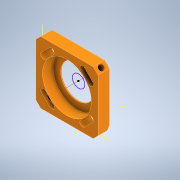
# Autodesk Inventor part: 20_Cube_Insert_Kinematic_Beautymirrormount_90_pro_v3
Saved by Autodesk Inventor 2022.3 (Build 263350000, 350)
## iProperties
Created: 2021-11-15
Part Number: 20_Cube_Insert_Kinematic_Beautymirrormount_90_pro_v3
Material: Generic
Document SubType Name: Modeling
Designer: diederichbenedict
Density: 1 g/cm^3
Appearance: Orange
Author: diederichbenedict
Autodesk Inventor part; units mm, degrees
ref_plane "YZ Plane" through (0, 0, 0) normal (1, 0, 0) x (0, 1, 0)
ref_plane "XY Plane" through (0, 0, 0) normal (0, 0, 1) x (1, 0, 0)
ref_plane "Work Plane1" through (0, 0, 2) normal (0, 0, 1) x (1, 0, 0)
sketch "Sketch1" plane through (0, 0, 2) normal (0, 0, 1) x (1, 0, 0)
  circle A0 centre (-37.0712, 14) radius 3.25 construction
  circle A1 centre (-9.0712, -14) radius 3.25 construction
  line L0 (-26.0712, -17.08) -> (-20.0712, -17.08) construction
  arc A2 (-20.0712, -17.08) -> (-20.0712, -14.08) centre (-20.0712, -15.58) ccw construction
  line L1 (-20.0712, -14.08) -> (-26.0712, -14.08) construction
  line L2 (-37.0712, -3) -> (-37.0712, 3) construction
  arc A3 (-37.0712, 3) -> (-40.0712, 3) centre (-38.5712, 3) ccw construction
  line L3 (-40.0712, 3) -> (-40.0712, -3) construction
  line L4 (-47.9712, -17) -> (-47.9712, 17) construction
  line L5 (-47.9712, 17) -> (-44.3964, 17) construction
  line L6 (-44.3964, 17) -> (-40.0712, 21.3252) construction
  line L7 (-40.0712, 21.3252) -> (-40.0712, 24.9) construction
  line L8 (-40.0712, 24.9) -> (-6.0712, 24.9) construction
  line L9 (-6.0712, 24.9) -> (-6.0712, 21.3252) construction
  line L10 (-6.0712, 21.3252) -> (-1.746, 17) construction
  line L11 (-1.746, 17) -> (1.8288, 17) construction
  line L12 (1.8288, 17) -> (1.8288, -17) construction
  line L13 (1.8288, -17) -> (-1.746, -17) construction
  line L14 (-1.746, -17) -> (-6.1126, -21.3666) construction
  line L15 (-6.1126, -21.3666) -> (-6.1126, -24.9) construction
  line L16 (-6.1126, -24.9) -> (-40.0712, -24.9) construction
  circle A4 centre (-37.0712, -14) radius 3.25 construction
  circle A5 centre (-23.0712, 0) radius 12.45 construction
  circle A6 centre (-23.0712, 0) radius 12.7 construction
  line L17 (-37.0712, 14) -> (-9.0712, 14) construction
  line L18 (-9.0712, 14) -> (-9.0712, -14) construction
  line L19 (-9.0712, -14) -> (-37.0712, -14) construction
  line L20 (-37.0712, -14) -> (-37.0712, 14) construction
  line L21 (-4.0712, -19) -> (-4.0712, 19)
  line L22 (-4.0712, 19) -> (-42.0712, 19)
  line L23 (-42.0712, 19) -> (-42.0712, -19)
  line L24 (-42.0712, -19) -> (-4.0712, -19)
  circle A7 centre (-23.0712, 0) radius 12.8
  circle A8 centre (-23.0712, 0) radius 3.25 projected
  line L25 (-40.0712, -24.9) -> (-40.0712, -21.3252) projected
  line L26 (-40.0712, -21.3252) -> (-44.3964, -17) projected
  line L27 (-44.3964, -17) -> (-47.9712, -17) projected
  arc A9 (-26.0712, -14.08) -> (-26.0712, -17.08) centre (-26.0712, -15.58) ccw projected
  arc A10 (-40.0712, -3) -> (-37.0712, -3) centre (-38.5712, -3) ccw projected
  circle A11 centre (-37.0712, -14) radius 3.25 projected
  point P0 (0, 0)
  point P1 (-21.8762, -3.0223)
  point P2 (-25.9925, 1.4242)
  dimension "d0" = 5
  dimension "d1" = 0.1
  constraints: 16 end point, 4 parallel, 2 perpendicular, 1 centre point, 1 horizontal, 3 other
  measures "d0" distance between parallel lines of L18 L21
  measures "d1" radial gap between concentric circles of A6 A7
extrude "Extrusion1" add sketch "Sketch1" along normal blind 6 contours L24 L23 L22 L21 | A7 | A8 | A11
sketch "Sketch2" plane through (0, 0, 2) normal (0, 0, -1) x (-1, 0, 0)
  circle A0 centre (23.0712, 0) radius 12.8 projected
  circle A1 centre (23.0712, 0) radius 8.5824
  point P0 (0, 0)
  constraints: 1 centre point
extrude "Extrusion2" add sketch "Sketch2" against normal blind 0.5
sketch "Sketch3" plane through (0, 0, 2) normal (0, 0, -1) x (-1, 0, 0)
  circle A0 centre (9.0712, -14) radius 1.45 construction
  circle A1 centre (9.0712, -14) radius 2.45
  circle A2 centre (37.0712, -14) radius 1.45 projected
  circle A3 centre (37.0712, -14) radius 1.95
  point P0 (0, 0)
  dimension "d8" = 1
  dimension "d10" = 0.5
  constraints: 2 centre point
  measures "d8" radial gap between concentric circles of A0 A1
  measures "d10" radial gap between concentric circles of A2 A3
sketch "Sketch5" plane through (0, 0, 2) normal (0, 0, -1) x (-1, 0, 0)
  arc A0 (20.0712, -14.08) -> (20.0712, -17.08) centre (20.0712, -15.58) ccw construction
  arc A1 (26.0712, -17.08) -> (26.0712, -14.08) centre (26.0712, -15.58) ccw construction
  line L0 (37.0712, 3) -> (37.0712, -3) projected
  arc A2 (37.0712, -3) -> (40.0712, -3) centre (38.5712, -3) ccw projected
  line L1 (40.0712, -3) -> (40.0712, 3) projected
  arc A3 (40.0712, 3) -> (37.0712, 3) centre (38.5712, 3) ccw projected
  line L2 (26.0712, -14.08) -> (20.0712, -14.08) construction
  arc A4 (20.0712, -14.08) -> (20.0712, -17.08) centre (20.0712, -15.58) ccw construction
  line L3 (20.0712, -17.08) -> (26.0712, -17.08) construction
  arc A5 (26.0712, -17.08) -> (26.0712, -14.08) centre (26.0712, -15.58) ccw construction
  circle A6 centre (37.0712, -14) radius 1.45 projected
  circle A7 centre (23.0712, 0) radius 1.45 projected
  circle A8 centre (9.0712, -14) radius 1.45 projected
  circle A9 centre (37.0712, 14) radius 1.45 projected
  line L4 (-1.8288, -17) -> (-1.8288, 17) projected
  line L5 (-1.8288, 17) -> (1.746, 17) projected
  line L6 (1.746, 17) -> (6.0712, 21.3252) projected
  line L7 (6.0712, 21.3252) -> (6.0712, 24.9) projected
  line L8 (6.0712, 24.9) -> (40.0712, 24.9) projected
  line L9 (40.0712, 24.9) -> (40.0712, 21.3252) projected
  line L10 (40.0712, 21.3252) -> (44.3964, 17) projected
  line L11 (44.3964, 17) -> (47.9712, 17) projected
  line L12 (47.9712, 17) -> (47.9712, -17) projected
  line L13 (44.3964, -17) -> (47.9712, -17) projected
  line L14 (40.0712, -21.3252) -> (44.3964, -17) projected
  line L15 (40.0712, -24.9) -> (40.0712, -21.3252) projected
  line L16 (6.1126, -24.9) -> (40.0712, -24.9) projected
  line L17 (6.1126, -24.9) -> (6.1126, -21.3666) projected
  line L18 (6.1126, -21.3666) -> (1.746, -17) projected
  line L19 (1.746, -17) -> (-1.8288, -17) projected
  line L20 (42.0712, -19) -> (4.0712, -19) projected
  arc A10 (7.0712, -3) -> (8.5712, -4.5) centre (8.5712, -3) ccw
  arc A11 (10.0712, 3) -> (8.5712, 4.5) centre (8.5712, 3) ccw
  line L21 (10.0712, 3) -> (10.0712, -3)
  line L22 (8.5712, 3) -> (8.5712, -3.1288) construction
  line L23 (7.0712, -3) -> (7.0712, 3)
  arc A12 (8.5712, 4.5) -> (7.0712, 3) centre (8.5712, 3) ccw
  arc A13 (8.5712, -4.5) -> (10.0712, -3) centre (8.5712, -3) ccw
  line L24 (4.0712, -19) -> (4.0712, 19) projected
  line L25 (42.0712, 19) -> (42.0712, -19) projected
  line L26 (4.0712, 19) -> (42.0712, 19) projected
  circle A14 centre (23.0712, 0) radius 16 construction
  arc A15 (20.0712, 16) -> (18.5712, 14.5) centre (20.0712, 14.5) ccw
  line L27 (26.0712, 14.5) -> (19.9423, 14.5) construction
  line L28 (20.0712, 16) -> (26.0712, 16)
  line L29 (26.0712, 13) -> (20.0712, 13)
  arc A16 (27.5712, 14.5) -> (26.0712, 16) centre (26.0712, 14.5) ccw
  arc A17 (26.0712, 13) -> (27.5712, 14.5) centre (26.0712, 14.5) ccw
  arc A18 (18.5712, 14.5) -> (20.0712, 13) centre (20.0712, 14.5) ccw
  arc A19 (39.0712, 3) -> (37.5712, 4.5) centre (37.5712, 3) ccw
  line L30 (37.5712, -3) -> (37.5712, 3.1288) construction
  line L31 (39.0712, 3) -> (39.0712, -3)
  line L32 (36.0712, -3) -> (36.0712, 3)
  arc A20 (37.5712, -4.5) -> (39.0712, -3) centre (37.5712, -3) ccw
  arc A21 (36.0712, -3) -> (37.5712, -4.5) centre (37.5712, -3) ccw
  arc A22 (37.5712, 4.5) -> (36.0712, 3) centre (37.5712, 3) ccw
  arc A23 (26.0712, -16) -> (27.5712, -14.5) centre (26.0712, -14.5) ccw
  line L33 (20.0712, -14.5) -> (26.2, -14.5) construction
  line L34 (26.0712, -16) -> (20.0712, -16)
  line L35 (20.0712, -13) -> (26.0712, -13)
  arc A24 (18.5712, -14.5) -> (20.0712, -16) centre (20.0712, -14.5) ccw
  arc A25 (20.0712, -13) -> (18.5712, -14.5) centre (20.0712, -14.5) ccw
  arc A26 (27.5712, -14.5) -> (26.0712, -13) centre (26.0712, -14.5) ccw
  arc A27 (13.8788, -13.435) -> (16.0001, -13.435) centre (14.9394, -12.3744) ccw
  circle A28 centre (23.0712, 0) radius 16 construction
  line L36 (11.7575, -7.0711) -> (16.0001, -11.3137)
  line L37 (13.8788, -13.435) -> (9.6361, -9.1924)
  line L38 (10.6968, -8.1317) -> (15.0305, -12.4655) construction
  arc A29 (36.5062, -7.0711) -> (34.3849, -7.0711) centre (35.4455, -8.1317) ccw
  arc A30 (9.6361, -7.0711) -> (9.6361, -9.1924) centre (10.6968, -8.1317) ccw
  arc A31 (11.7575, -7.0711) -> (9.6361, -7.0711) centre (10.6968, -8.1317) ccw
  arc A32 (16.0001, -13.435) -> (16.0001, -11.3137) centre (14.9394, -12.3744) ccw
  arc A33 (9.6361, 9.1924) -> (9.6361, 7.0711) centre (10.6968, 8.1317) ccw
  line L39 (14.9394, 12.3744) -> (10.6057, 8.0406) construction
  arc A34 (16.0001, 11.3137) -> (16.0001, 13.435) centre (14.9394, 12.3744) ccw
  arc A35 (16.0001, 13.435) -> (13.8788, 13.435) centre (14.9394, 12.3744) ccw
  line L40 (16.0001, 11.3137) -> (11.7575, 7.0711)
  line L41 (9.6361, 9.1924) -> (13.8788, 13.435)
  arc A36 (9.6361, 7.0711) -> (11.7575, 7.0711) centre (10.6968, 8.1317) ccw
  line L42 (34.3849, 7.0711) -> (30.1422, 11.3137)
  arc A37 (34.3849, 7.0711) -> (36.5062, 7.0711) centre (35.4455, 8.1317) ccw
  arc A38 (30.1422, 13.435) -> (30.1422, 11.3137) centre (31.2029, 12.3744) ccw
  line L43 (35.4455, 8.1317) -> (31.1118, 12.4655) construction
  arc A39 (32.2636, 13.435) -> (30.1422, 13.435) centre (31.2029, 12.3744) ccw
  line L44 (32.2636, 13.435) -> (36.5062, 9.1924)
  arc A40 (36.5062, 7.0711) -> (36.5062, 9.1924) centre (35.4455, 8.1317) ccw
  line L45 (31.2029, -12.3744) -> (35.5366, -8.0406) construction
  line L46 (30.1422, -11.3137) -> (34.3849, -7.0711)
  arc A41 (30.1422, -11.3137) -> (30.1422, -13.435) centre (31.2029, -12.3744) ccw
  line L47 (36.5062, -9.1924) -> (32.2636, -13.435)
  arc A42 (30.1422, -13.435) -> (32.2636, -13.435) centre (31.2029, -12.3744) ccw
  arc A43 (36.5062, -9.1924) -> (36.5062, -7.0711) centre (35.4455, -8.1317) ccw
  point P0 (0, 0)
  point P1 (40.0712, -3)
  point P2 (4.0712, 0)
  point P3 (7.0712, 0)
  point P4 (23.0712, 16)
  point P5 (39.0712, 0)
  point P6 (23.0712, -16)
  point P7 (11.7575, -11.3137)
  point P8 (13.8788, -9.1924)
  point P9 (11.7575, 11.3137)
  point P10 (34.3849, 11.3137)
  point P11 (34.3849, -11.3137)
  point P12 (11.7575, 11.3137)
  point P13 (34.3849, -11.3137)
  point P14 (34.3849, 11.3137)
  point P15 (13.8788, -9.1924)
  dimension "d133" = 360
  dimension "d144" = 360
  dimension "d240" = 32
  dimension "d139" = 1.5
  dimension "d140" = 1.5
  dimension "d141" = 3
  dimension "d234" = 3
  dimension "d235" = 9
  dimension "d238" = 360
  dimension "d280" = 1.5
  dimension "d281" = 1.5
  dimension "d282" = 3
  dimension "d283" = 3
  dimension "d284" = 9
  dimension "d285" = 32
  constraints: 69 point on circle, 48 end point, 33 centre point, 16 point on line, 12 coincident, 7 midpoint, 7 parallel, 4 vertical alignment, 1 horizontal alignment, 79 other
  measures "d139" radius of A11
  measures "d140" radius of A10
  measures "d141" distance between parallel lines of L21 L23
  measures "d234" distance from line of point (7.071, 0) L21
  measures "d235" distance of A10.end A11.end
  measures "d280" radius of A31
  measures "d281" radius of A27
  measures "d282" distance between parallel lines of L36 L37
  measures "d283" distance from line of A28.start L36
  measures "d284" distance of A32.start A31.end
  measures "d285" diameter of A28
extrude "Extrusion5" cut sketch "Sketch5" against normal blind 8 contours L37 A30 A31 L36 A32 A27 | A43 L47 A42 A41 L46 A29 | L41 A35 A34 L40 A36 A33 | L42 A38 A39 L44 A40 A37
sketch "Sketch6" plane through (-42.0712, -19, 8) normal (0, -1, 0) x (1, 0, 0)
  line L0 (0, -6) -> (38, -6) projected
  line L1 (38, -6) -> (38, 0) projected
  line L2 (0, 0) -> (38, 0) projected
  line L3 (0, -6) -> (0, 0) projected
  line L4 (31.8, 0) -> (31.8, 0) projected
  circle A0 centre (19, -3.5) radius 1.45
  point P0 (42.0712, -8)
  point P1 (4.5, 0)
  dimension "d34" = 2.9
  dimension "d126" = 2.5
  constraints: 1 centre point
  measures "d34" diameter of A0
  measures "d126" distance from line of L0 A0.centre
extrude "Extrusion6" [suppressed]
pattern_circular "Circular Pattern1" [suppressed]
chamfer "Chamfer1" distance 3 angle 45 4 edges at (-42.0712, 19, 5) (-4.0712, 19, 5) (-4.0712, -19, 5) (-42.0712, -19, 5)
sketch "Sketch13" plane through (0, 0, 2) normal (0, 0, -1) x (-1, 0, 0)
  circle A0 centre (23.0712, 0) radius 10.0484
  line L0 (42.0712, 16) -> (42.0712, -16) projected
  line L1 (39.0712, -19) -> (7.0712, -19) projected
  circle A1 centre (23.0712, 0) radius 3.25
  point P0 (0, 0)
  point P1 (42.0712, 0)
  point P2 (23.0712, -19)
  constraints: 2 centre point, 2 midpoint, 1 coincident, 1 horizontal alignment, 1 vertical alignment
hole "Hole1" at (-37.0712, -14, 2) direction (0, 0, 1) diameter 4 depth 0.1 tip angle 115
sketch "Sketch4" plane through (-4.0712, -19, 2) normal (1, 0, 0) x (0, 0, -1)
  line L0 (2, 4.45) -> (6, 4.45)
  line L1 (2, 1.55) -> (6, 1.55)
  line L2 (0, 0) -> (0, 38) projected
  arc A0 (2, 19) -> (2, 19) centre (1.5, 4.4206) ccw projected
  line L3 (-1.3741, 5) -> (-0.1, 7) projected
  line L4 (-1.3741, 5) -> (-0.1, 3) projected
  line L5 (-0.1, 7) -> (0.6045, 7)
  line L6 (0.6045, 7) -> (0.6045, 3)
  line L7 (0.6045, 3) -> (-0.1, 3)
  line L8 (-0.1, 3) -> (-0.1, 7)
  constraints: 12 end point, 3 horizontal, 2 parallel, 1 perpendicular, 4 other
extrude "Extrusion4" cut sketch "Sketch4" against normal blind 8 contours L7 L8 L5 L2 | L2 L5 L6 L7 | L4 L3 L8
sketch "Sketch9" plane through (-39.0712, 19, 2) normal (0, 1, 0) x (1, 0, 0)
  line L0 (35.8594, -6) -> (35.8594, -4)
  line L1 (35.8594, -4) -> (-5.4569, -4)
  line L2 (-5.4569, -4) -> (-5.4569, -6)
  line L3 (-5.4569, -6) -> (35.8594, -6)
  line L4 (32, -6) -> (0, -6) projected
  point P0 (39.0712, 2)
  dimension "d51" = 2
  constraints: 8 end point, 2 parallel, 1 collinear, 1 perpendicular, 1 vertical
  measures "d51" distance between parallel lines of L1 L3
extrude "Extrusion9" [suppressed]
sketch "Sketch11" plane through (0, 0, 2) normal (0, 0, -1) x (-1, 0, 0)
  circle A0 centre (23.0712, 0) radius 3.25 projected
  line L0 (12.0712, -16) -> (4.0712, -16) projected
  line L1 (7.0712, -19) -> (4.0712, -16) projected
  line L2 (39.0712, -19) -> (7.0712, -19) projected
  line L3 (42.0712, -16) -> (39.0712, -19) projected
  line L4 (42.0712, 16) -> (42.0712, -16) projected
  line L5 (39.0712, 19) -> (42.0712, 16) projected
  line L6 (7.0712, 19) -> (39.0712, 19) projected
  line L7 (4.0712, 16) -> (7.0712, 19) projected
  line L8 (4.0712, -12) -> (4.0712, 16) projected
  line L9 (4.0712, -12) -> (12.0712, -12) projected
  line L10 (12.0712, -12) -> (12.0712, -16) projected
  circle A1 centre (37.0712, -14) radius 2 projected
  circle A2 centre (23.0712, 0) radius 3.25 projected
  line L11 (4.0712, -12) -> (4.0712, 16) projected
  circle A3 centre (13.1721, 17.5) radius 1
  circle A4 centre (33.6721, 11) radius 1
  circle A5 centre (18.1721, -10.5) radius 1
  circle A6 centre (33.6721, 11) radius 0.9
  circle A7 centre (13.1721, 17.5) radius 0.9
  circle A8 centre (18.1721, -10.5) radius 0.9
  circle A9 centre (23.0712, 0) radius 7.071
  point P0 (0, 0)
  point P1 (0, 0)
  dimension "d57" = 1.8
  dimension "d58" = 1.8
  dimension "d59" = 1.8
  constraints: 7 centre point, 3 coincident
  measures "d57" diameter of A6
  measures "d58" diameter of A7
  measures "d59" diameter of A8
extrude "Extrusion10" [suppressed]
sketch "Sketch12" plane through (0, 0, 8) normal (0, 0, 1) x (1, 0, 0)
  line L0 (-32.0962, 9.025) -> (-14.0462, 9.025) construction
  line L1 (-14.0462, 9.025) -> (-14.0462, -9.025) construction
  line L2 (-14.0462, -9.025) -> (-32.0962, -9.025) construction
  line L3 (-32.0962, -9.025) -> (-32.0962, 9.025) construction
  line L4 (-7.0712, 19) -> (-39.0712, 19) projected
  line L5 (-4.0712, -16) -> (-4.0712, 16) projected
  circle A0 centre (-23.0712, 0) radius 12.8
  point P0 (0, 0)
  point P1 (-23.0712, 9.025)
  point P2 (-23.0712, 19)
  point P3 (-14.0462, 0)
  point P4 (-4.0712, 0)
  dimension "d62" = 18.05
  dimension "d63" = 18.05
  dimension "d205" = 25.6
  constraints: 8 end point, 4 midpoint, 2 parallel, 1 centre point, 1 horizontal, 1 horizontal alignment, 1 perpendicular, 1 vertical alignment
  measures "d62" distance of L0.start L0.end
  measures "d63" distance of L0.end L1.end
  measures "d205" diameter of A0
extrude "Extrusion11" cut sketch "Sketch12" against normal blind 6
sketch "Sketch14" plane through (0, 0, 8) normal (0, 0, 1) x (1, 0, 0)
  line L0 (-39.0712, -19) -> (-42.0712, -16) projected
  line L1 (-39.0712, -19) -> (-7.0712, -19) projected
  line L2 (-4.0712, -16) -> (-7.0712, -19) projected
  line L3 (-4.0712, -16) -> (-4.0712, 16) projected
  line L4 (-7.0712, 19) -> (-4.0712, 16) projected
  line L5 (-7.0712, 19) -> (-39.0712, 19) projected
  line L6 (-42.0712, 16) -> (-39.0712, 19) projected
  line L7 (-42.0712, 16) -> (-42.0712, -16) projected
  line L8 (-36.8212, 16.3) -> (-9.3212, 16.3)
  line L9 (-9.3212, 16.3) -> (-6.7712, 13.75)
  line L10 (-6.7712, 13.75) -> (-6.7712, -13.75)
  line L11 (-6.7712, -13.75) -> (-9.3212, -16.3)
  line L12 (-9.3212, -16.3) -> (-36.8212, -16.3)
  line L13 (-36.8212, -16.3) -> (-39.3712, -13.75)
  line L14 (-39.3712, -13.75) -> (-39.3712, 13.75)
  line L15 (-39.3712, 13.75) -> (-36.8212, 16.3)
  line L16 (-7.0712, 19) -> (-39.0712, 19) projected
  line L17 (-7.0712, 19) -> (-4.0712, 16) projected
  line L18 (-4.0712, -16) -> (-7.0712, -19) projected
  line L19 (-4.0712, -16) -> (-4.0712, 16) projected
  line L20 (-39.0712, -19) -> (-7.0712, -19) projected
  line L21 (-39.0712, -19) -> (-42.0712, -16) projected
  line L22 (-42.0712, 16) -> (-42.0712, -16) projected
  line L23 (-42.0712, 16) -> (-39.0712, 19) projected
  point P0 (-23.0712, 16.3)
  point P1 (-23.0712, 19)
  point P2 (-23.0712, -16.3)
  point P3 (-6.7712, 0)
  point P4 (-4.0712, 0)
  point P5 (-39.3712, 0)
  point P6 (-42.0712, 0)
  point P7 (-8.0462, -15.025)
  point P8 (-38.0962, 15.025)
  point P9 (-38.0962, -15.025)
  point P10 (-8.0462, 15.025)
  dimension "d190" = 27.5
  dimension "d194" = 2.7
  dimension "d195" = 2.7
  dimension "d196" = 2.7
  dimension "d197" = 2.7
  dimension "d198" = 27.5
  dimension "d199" = 27.5
  dimension "d200" = 27.5
  dimension "d201" = 3.6062
  dimension "d202" = 3.6062
  dimension "d203" = 3.6062
  dimension "d204" = 3.6062
  constraints: 16 end point, 11 midpoint, 10 parallel, 3 perpendicular, 2 horizontal alignment, 2 vertical alignment, 1 horizontal
  measures "d190" distance of L8.start L8.end
  measures "d194" distance between parallel lines of L8 L5
  measures "d195" distance between parallel lines of L3 L10
  measures "d196" distance between parallel lines of L1 L12
  measures "d197" distance between parallel lines of L7 L14
  measures "d198" distance of L9.end L10.end
  measures "d199" distance of L13.end L14.end
  measures "d200" distance of L11.end L12.end
  measures "d201" distance of L14.end L8.start
  measures "d202" distance of L8.end L9.end
  measures "d203" distance of L10.end L11.end
  measures "d204" distance of L12.end L13.end
extrude "Extrusion12" cut sketch "Sketch14" against normal blind 10 contours L8 L9 L10 L11 L12 L13 L14 L15 keep common part
sketch "Sketch16" plane through (0, 0, 2) normal (0, 0, -1) x (-1, 0, 0)
  circle A0 centre (23.0712, 0) radius 12.8
  circle A1 centre (23.0712, 0) radius 8.8
  point P0 (0, 0)
  point P1 (14.0462, -9.025)
  dimension "d206" = 25.6
  dimension "d207" = 4
  constraints: 2 centre point, 1 coincident
  measures "d206" diameter of A0
  measures "d207" radial gap between concentric circles of A1 A0
extrude "Extrusion14" add sketch "Sketch16" against normal blind 0.5
sketch "Sketch17" plane through (-36.4185, -16.7027, 8) normal (-0.7071, -0.7071, 0) x (-0.7071, 0.7071, 0)
  line L0 (0.3726, 6) -> (4.3726, 6) projected
  point P0 (-13.9412, 8)
  point P1 (3.7506, 6)
sketch "Sketch18" plane through (0, 0, 8) normal (0, 0, 1) x (1, 0, 0)
  circle A0 centre (-23.0712, 0) radius 12.8 projected
  circle A1 centre (-23.0712, 0) radius 12.8 projected
  line L0 (-20.0712, 14.5) -> (-26.0712, 14.5) construction
  line L1 (-20.0712, 16) -> (-26.0712, 16)
  line L2 (-26.0712, 13) -> (-20.0712, 13)
  arc A2 (-20.0712, 13) -> (-20.0712, 16) centre (-20.0712, 14.5) ccw
  arc A3 (-26.0712, 16) -> (-26.0712, 13) centre (-26.0712, 14.5) ccw
  arc A4 (-10.0712, -3) -> (-7.0712, -3) centre (-8.5712, -3) ccw projected
  line L3 (-8.5712, -3) -> (-8.5712, 3) construction
  line L4 (-10.0712, -3) -> (-10.0712, 3)
  line L5 (-7.0712, 3) -> (-7.0712, -3)
  arc A5 (-10.0712, -3) -> (-7.0712, -3) centre (-8.5712, -3) ccw
  arc A6 (-7.0712, 3) -> (-10.0712, 3) centre (-8.5712, 3) ccw
  line L6 (-20.0712, -14.5) -> (-26.0712, -14.5) construction
  line L7 (-20.0712, -13) -> (-26.0712, -13)
  line L8 (-26.0712, -16) -> (-20.0712, -16)
  arc A7 (-20.0712, -16) -> (-20.0712, -13) centre (-20.0712, -14.5) ccw
  arc A8 (-26.0712, -13) -> (-26.0712, -16) centre (-26.0712, -14.5) ccw
  line L9 (-37.5712, -3) -> (-37.5712, 3) construction
  line L10 (-39.0712, -3) -> (-39.0712, 3)
  line L11 (-36.0712, 3) -> (-36.0712, -3)
  arc A9 (-39.0712, -3) -> (-36.0712, -3) centre (-37.5712, -3) ccw
  arc A10 (-36.0712, 3) -> (-39.0712, 3) centre (-37.5712, 3) ccw
  line L12 (-20.0712, -14.5) -> (-26.0712, -14.5) construction
  line L13 (-20.0712, -13.25) -> (-26.0712, -13.25)
  line L14 (-26.0712, -15.75) -> (-20.0712, -15.75)
  arc A11 (-20.0712, -15.75) -> (-20.0712, -13.25) centre (-20.0712, -14.5) ccw
  arc A12 (-26.0712, -13.25) -> (-26.0712, -15.75) centre (-26.0712, -14.5) ccw
  line L15 (-8.5712, -3) -> (-8.5712, 3) construction
  line L16 (-9.8212, -3) -> (-9.8212, 3)
  line L17 (-7.3212, 3) -> (-7.3212, -3)
  arc A13 (-9.8212, -3) -> (-7.3212, -3) centre (-8.5712, -3) ccw
  arc A14 (-7.3212, 3) -> (-9.8212, 3) centre (-8.5712, 3) ccw
  line L18 (-20.0712, 14.5) -> (-26.0712, 14.5) construction
  line L19 (-20.0712, 15.75) -> (-26.0712, 15.75)
  line L20 (-26.0712, 13.25) -> (-20.0712, 13.25)
  arc A15 (-20.0712, 13.25) -> (-20.0712, 15.75) centre (-20.0712, 14.5) ccw
  arc A16 (-26.0712, 15.75) -> (-26.0712, 13.25) centre (-26.0712, 14.5) ccw
  line L21 (-37.5712, 3) -> (-37.5712, -3) construction
  line L22 (-38.8212, 3) -> (-38.8212, -3)
  line L23 (-36.3212, -3) -> (-36.3212, 3)
  arc A17 (-36.3212, 3) -> (-38.8212, 3) centre (-37.5712, 3) ccw
  arc A18 (-38.8212, -3) -> (-36.3212, -3) centre (-37.5712, -3) ccw
  line L24 (-10.6968, 8.1317) -> (-14.9394, 12.3744) construction
  line L25 (-9.6361, 9.1924) -> (-13.8788, 13.435)
  line L26 (-16.0001, 11.3137) -> (-11.7575, 7.0711)
  arc A19 (-11.7575, 7.0711) -> (-9.6361, 9.1924) centre (-10.6968, 8.1317) ccw
  arc A20 (-13.8788, 13.435) -> (-16.0001, 11.3137) centre (-14.9394, 12.3744) ccw
  line L27 (-14.9394, -12.3744) -> (-10.6968, -8.1317) construction
  line L28 (-16.0001, -11.3137) -> (-11.7575, -7.0711)
  line L29 (-9.6361, -9.1924) -> (-13.8788, -13.435)
  arc A21 (-16.0001, -11.3137) -> (-13.8788, -13.435) centre (-14.9394, -12.3744) ccw
  arc A22 (-9.6361, -9.1924) -> (-11.7575, -7.0711) centre (-10.6968, -8.1317) ccw
  line L30 (-31.2029, -12.3744) -> (-35.4455, -8.1317) construction
  line L31 (-30.1422, -11.3137) -> (-34.3849, -7.0711)
  line L32 (-36.5062, -9.1924) -> (-32.2636, -13.435)
  arc A23 (-32.2636, -13.435) -> (-30.1422, -11.3137) centre (-31.2029, -12.3744) ccw
  arc A24 (-34.3849, -7.0711) -> (-36.5062, -9.1924) centre (-35.4455, -8.1317) ccw
  line L33 (-35.4455, 8.1317) -> (-31.2029, 12.3744) construction
  line L34 (-36.5062, 9.1924) -> (-32.2636, 13.435)
  line L35 (-30.1422, 11.3137) -> (-34.3849, 7.0711)
  arc A25 (-36.5062, 9.1924) -> (-34.3849, 7.0711) centre (-35.4455, 8.1317) ccw
  arc A26 (-30.1422, 11.3137) -> (-32.2636, 13.435) centre (-31.2029, 12.3744) ccw
  line L36 (-31.2029, -12.3744) -> (-35.4455, -8.1317) construction
  line L37 (-30.319, -11.4905) -> (-34.5617, -7.2478)
  line L38 (-36.3294, -9.0156) -> (-32.0868, -13.2583)
  arc A27 (-32.0868, -13.2583) -> (-30.319, -11.4905) centre (-31.2029, -12.3744) ccw
  arc A28 (-34.5617, -7.2478) -> (-36.3294, -9.0156) centre (-35.4455, -8.1317) ccw
  line L39 (-14.9394, -12.3744) -> (-10.6968, -8.1317) construction
  line L40 (-15.8233, -11.4905) -> (-11.5807, -7.2478)
  line L41 (-9.8129, -9.0156) -> (-14.0556, -13.2583)
  arc A29 (-15.8233, -11.4905) -> (-14.0556, -13.2583) centre (-14.9394, -12.3744) ccw
  arc A30 (-9.8129, -9.0156) -> (-11.5807, -7.2478) centre (-10.6968, -8.1317) ccw
  line L42 (-10.6968, 8.1317) -> (-14.9394, 12.3744) construction
  line L43 (-9.8129, 9.0156) -> (-14.0556, 13.2583)
  line L44 (-15.8233, 11.4905) -> (-11.5807, 7.2478)
  arc A31 (-11.5807, 7.2478) -> (-9.8129, 9.0156) centre (-10.6968, 8.1317) ccw
  arc A32 (-14.0556, 13.2583) -> (-15.8233, 11.4905) centre (-14.9394, 12.3744) ccw
  line L45 (-31.2029, 12.3744) -> (-35.4455, 8.1317) construction
  line L46 (-32.0868, 13.2583) -> (-36.3294, 9.0156)
  line L47 (-34.5617, 7.2478) -> (-30.319, 11.4905)
  arc A33 (-30.319, 11.4905) -> (-32.0868, 13.2583) centre (-31.2029, 12.3744) ccw
  arc A34 (-36.3294, 9.0156) -> (-34.5617, 7.2478) centre (-35.4455, 8.1317) ccw
  circle A35 centre (-23.0712, 0) radius 3.6722
  point P0 (-23.0712, 14.5)
  point P1 (-8.5712, 0)
  point P2 (-23.0712, -14.5)
  point P3 (-37.5712, 0)
  point P4 (-23.0712, -14.5)
  point P5 (-8.5712, 0)
  point P6 (-23.0712, 14.5)
  point P7 (-37.5712, 0)
  point P8 (-12.8181, 10.253)
  point P9 (-12.8181, -10.253)
  point P10 (-33.3242, -10.253)
  point P11 (-33.3242, 10.253)
  point P12 (-33.3242, -10.253)
  point P13 (-12.8181, -10.253)
  point P14 (-12.8181, 10.253)
  point P15 (-33.3242, 10.253)
  dimension "d218" = 360
  dimension "d263" = 14.5
  dimension "d264" = 14.5
  dimension "d265" = 14.5
  dimension "d266" = 14.5
  dimension "d267" = 14.5
  dimension "d268" = 14.5
  dimension "d269" = 14.5
  constraints: 128 end point, 64 point on circle, 64 tangent, 33 centre point, 18 parallel, 16 midpoint, 8 perpendicular, 2 horizontal alignment, 1 horizontal, 1 vertical, 1 vertical alignment, 1 other
  measures "d263" distance of A0.centre point (-23.071, 14.5)
  measures "d264" distance of A1.centre point (-23.071, -14.5)
  measures "d265" distance of A1.centre point (-8.571, 0)
  measures "d266" distance of A35.centre point (-33.324, 10.253)
  measures "d267" distance of A35.centre point (-12.818, 10.253)
  measures "d268" distance of point (-12.818, -10.253) A35.centre
  measures "d269" distance of A35.centre point (-33.324, -10.253)
extrude "Extrusion16" [suppressed]
sketch "Sketch20" plane through (-9.3212, 16.3, 2) normal (0.7071, 0.7071, 0) x (-0.7071, 0.7071, 0)
  circle A0 centre (-1.8031, 3) radius 1.45
  line L0 (-3.6062, 6) -> (-3.6062, 0) projected
  line L1 (0, 6) -> (-3.6062, 6) projected
  point P0 (-18.1169, -2)
  point P1 (-3.6062, 3)
  point P2 (-1.8031, 6)
  dimension "d286" = 2.9
  constraints: 2 midpoint, 1 centre point, 1 horizontal alignment, 1 vertical alignment
  measures "d286" diameter of A0
extrude "Extrusion18" cut sketch "Sketch20" against normal up to surface (5.2486 mm away)
pattern_circular "Circular Pattern4" count 4 over 360 about axis through (-23.0712, 0, 2) along (0, 0, -1) of "Extrusion18"
equation "\"d63\" = d62"
body "Solid1"
